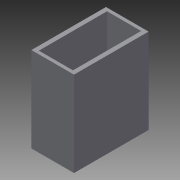
# Autodesk Inventor part: atmos-pressure-end
Saved by Autodesk Inventor 2014 SP2 (Build 180246200, 246)
## iProperties
Created: 2014-06-30
Part Number: atmos-pressure-end
Material: Generic
Document SubType Name: Modeling
Designer: pjb08r
Density: 1 g/cm^3
Appearance: Default
Author: pjb08r
Autodesk Inventor part; units mm, degrees
ref_plane "YZ Plane" through (0, 0, 0) normal (1, 0, 0) x (0, 1, 0)
ref_plane "XZ Plane" through (0, 0, 0) normal (0, 1, 0) x (-1, 0, 0)
ref_plane "XY Plane" through (0, 0, 0) normal (0, 0, 1) x (1, 0, 0)
sketch "Sketch1" plane through (0, 0, 0) normal (0, 0, 1) x (1, 0, 0)
  line L0 (-10, -17.5) -> (10, -17.5)
  line L1 (10, -17.5) -> (10, 17.5)
  line L2 (10, 17.5) -> (-10, 17.5)
  line L3 (-10, 17.5) -> (-10, -17.5)
  line L4 (-10, -17.5) -> (10, 17.5) construction
  line L5 (10, -17.5) -> (-10, 17.5) construction
  point P0 (0, 0)
  dimension "d0" = 20
  dimension "d1" = 35
  constraints: 12 end point, 2 midpoint, 2 parallel, 1 horizontal, 1 perpendicular
  measures "d0" distance of L2.end L1.end
  measures "d1" distance of L1.end L0.end
extrude "Extrusion1" add sketch "Sketch1" along normal blind 40
sketch "Sketch2" plane through (0, 0, 40) normal (0, 0, 1) x (1, 0, 0)
  line L0 (-8, -16) -> (8, -16)
  line L1 (8, -16) -> (8, 16)
  line L2 (8, 16) -> (-8, 16)
  line L3 (-8, 16) -> (-8, -16)
  point P0 (0, 0)
  dimension "d4" = 16
  dimension "d5" = 32
  constraints: 8 end point, 2 parallel, 1 horizontal, 1 perpendicular
  measures "d4" distance of L2.end L1.end
  measures "d5" distance of L1.end L0.end
extrude "Extrusion2" cut sketch "Sketch2" against normal blind 30
sketch "Sketch3" plane through (0, 0, 10) normal (0, 0, 1) x (1, 0, 0)
  line L0 (8, -16) -> (-8, -16) projected
  line L1 (8, 16) -> (8, -16) projected
  line L2 (-8, 16) -> (8, 16) projected
  line L3 (-8, -16) -> (-8, 16) projected
  point P0 (0, 0)
sketch "Sketch4" plane through (0, 0, 10) normal (0, 0, 1) x (1, 0, 0)
  circle A0 centre (0, 6) radius 2.5
  point P0 (0, 0)
  dimension "d8" = 5
  constraints: 1 centre point
  measures "d8" diameter of A0
hole "Hole1" at (0, 6, 10) direction (0, 0, -1) diameter 5 end through all
body "Solid1"
